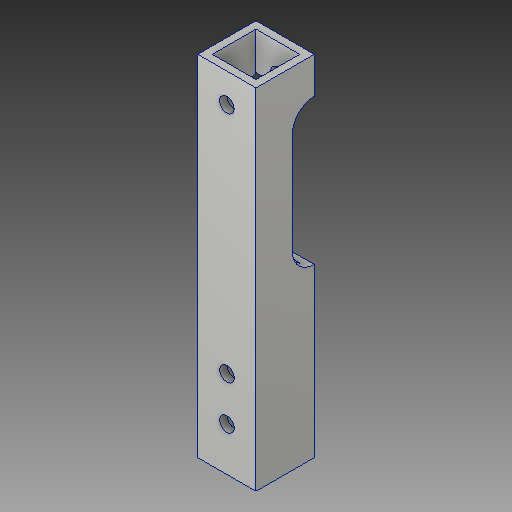
# Autodesk Inventor part: 6x1x1x0125 tube
Saved by Autodesk Inventor 2017 (Build 210142000, 142)
## iProperties
Created: 2016-10-01
Part Number: 6x1x1x0125 tube
Material: Aluminum 6061
Document SubType Name: Modeling
Designer: 15102898
Density: 2.7 g/cm^3
Appearance: Aluminum - Flat
Author: 15102898
Autodesk Inventor part; units mm, degrees
ref_plane "YZ Plane" through (0, 0, 0) normal (1, 0, 0) x (0, 1, 0)
ref_plane "XZ Plane" through (0, 0, 0) normal (0, 1, 0) x (-1, 0, 0)
ref_plane "XY Plane" through (0, 0, 0) normal (0, 0, 1) x (1, 0, 0)
sketch "Sketch1" plane through (0, 0, 0) normal (0, 1, 0) x (-1, 0, 0)
  line L0 (0, 0) -> (25.4, 0)
  line L1 (25.4, 0) -> (25.4, 25.4)
  line L2 (25.4, 25.4) -> (0, 25.4)
  line L3 (0, 25.4) -> (0, 0)
  line L4 (3.175, 22.225) -> (22.225, 22.225)
  line L5 (22.225, 22.225) -> (22.225, 3.175)
  line L6 (22.225, 3.175) -> (3.175, 3.175)
  line L7 (3.175, 3.175) -> (3.175, 22.225)
  dimension "d0" = 25.4
  dimension "d1" = 25.4
  dimension "d2" = 3.175
  dimension "d3" = 3.175
  dimension "d4" = 3.175
  dimension "d5" = 3.175
  constraints: 16 end point, 4 parallel, 2 horizontal, 2 perpendicular
  measures "d0" distance of L2.end L1.end
  measures "d1" distance of L2.end L0.start
  measures "d2" distance between parallel lines of L1 L5
  measures "d3" distance between parallel lines of L0 L6
  measures "d4" distance between parallel lines of L3 L7
  measures "d5" distance between parallel lines of L2 L4
extrude "Extrusion1" add sketch "Sketch1" along normal blind 152.4
sketch "Sketch2" plane through (-25.4, 0, 25.4) normal (0, 0, 1) x (1, 0, 0)
  circle A0 centre (12.7, 139.7) radius 3.175
  line L0 (0, 152.4) -> (25.4, 152.4) projected
  line L1 (0, 0) -> (0, 152.4) projected
  point P0 (25.4, 0)
  dimension "d8" = 6.35
  dimension "d9" = 12.7
  dimension "d10" = 12.7
  constraints: 1 centre point
  measures "d8" diameter of A0
  measures "d9" distance from line of A0.centre L0
  measures "d10" distance from line of L1 A0.centre
extrude "Extrusion2" cut sketch "Sketch2" against normal blind 152.4
sketch "Sketch3" plane through (-25.4, 0, 0) normal (-1, 0, 0) x (0, 0, 1)
  line L0 (0, 0) -> (0, 152.4) projected
  line L1 (0, 127) -> (0, 82.55) construction
  line L2 (-9.525, 127) -> (-9.525, 82.55)
  line L3 (9.525, 82.55) -> (9.525, 127)
  arc A0 (9.525, 127) -> (-9.525, 127) centre (0, 127) ccw
  arc A1 (-9.525, 82.55) -> (9.525, 82.55) centre (0, 82.55) ccw
  line L4 (0, 152.4) -> (25.4, 152.4) projected
  line L5 (0, 0) -> (25.4, 0) projected
  point P0 (0, 104.775)
  dimension "d13" = 44.45
  dimension "d14" = 19.05
  dimension "d15" = 25.4
  dimension "d16" = 82.55
  constraints: 8 end point, 4 point on circle, 4 tangent, 2 centre point, 2 point on line, 1 midpoint, 1 parallel
  measures "d13" distance of L1.start L1.end
  measures "d14" diameter of A1
  measures "d15" distance from line of L4 L1.start
  measures "d16" distance from line of L5 L1.end
extrude "Extrusion3" cut sketch "Sketch3" against normal blind 25.4
sketch "Sketch4" plane through (0, 0, 0) normal (0, 0, -1) x (-1, 0, 0)
  line L0 (0, 0) -> (25.4, 0) projected
  line L1 (25.4, 0) -> (25.4, 73.025) projected
  circle A0 centre (12.7, 38.1) radius 3.175
  circle A1 centre (12.7, 19.05) radius 3.175
  dimension "d19" = 19.05
  dimension "d20" = 12.7
  dimension "d21" = 12.7
  dimension "d22" = 19.05
  dimension "d23" = 6.35
  dimension "d24" = 6.35
  constraints: 2 centre point, 2 coincident
  measures "d19" distance from line of L0 point (12.7, 19.05)
  measures "d20" distance from line of L1 point (12.7, 19.05)
  measures "d21" distance from line of L1 point (12.7, 38.1)
  measures "d22" distance of point (12.7, 19.05) point (12.7, 38.1)
  measures "d23" diameter of A0
  measures "d24" diameter of A1
extrude "Extrusion4" cut sketch "Sketch4" against normal blind 25.4
equation "\"d4\" = d2"
equation "\"d5\" = d3"
body "Solid1"
